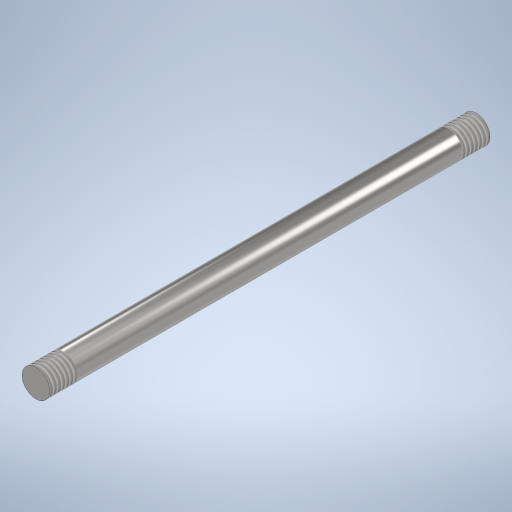
# Autodesk Inventor part: verbinder2
Saved by Autodesk Inventor 2024.4 (Build 284460000, 460)
## iProperties
Created: 2026-01-07
Part Number: verbinder2
Material: Edelstahl
Description: verbinder2
Document SubType Name: Modeling
Designer: Philf
Density: 8 g/cm^3
Appearance: Halbpoliert
Mass: 100.531 g
Surface Area: 51.8363 cm^2
Volume: 12.5664 cm^3
Sending System: SolidWorks 2024
Preprocessor: SwSTEP 2.0
Revision Number: ANY
Autodesk Inventor part; units mm, degrees
ref_plane "YZ Plane" through (0, 0, 0) normal (1, 0, 0) x (0, 1, 0)
ref_plane "XZ Plane" through (0, 0, 0) normal (0, 1, 0) x (-1, 0, 0)
ref_plane "XY Plane" through (0, 0, 0) normal (0, 0, 1) x (1, 0, 0)
sketch "Skizze1" plane through (0, 0, 0) normal (0, 1, 0) x (-1, 0, 0)
  circle A0 centre (0, 0) radius 5
  dimension "d0" = 10
  constraints: 1 centre point, 1 coincident
  measures "d0" diameter of A0
extrude "Extrusion1" add sketch "Skizze1" along normal blind 160
thread "Gewinde1" size "M10x1.5" class "6g" standard "ANSI Metric M Profile" length 10
thread "Gewinde2" size "M10x1.5" class "6g" standard "ANSI Metric M Profile" length 10
